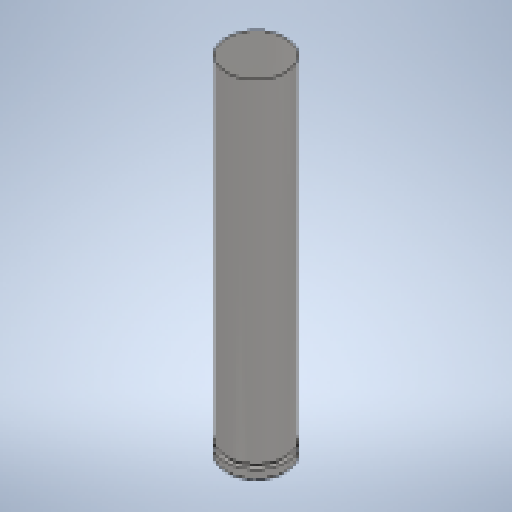
# Autodesk Inventor part: SHAFT
Saved by Autodesk Inventor 2023.2 (Build 272271000, 271)
## iProperties
Created: 2024-01-31
Part Number: SHAFT
Material: Stainless Steel
Document SubType Name: Modeling
Designer: Nathan Cai
Density: 8 g/cm^3
Appearance: Semi-Polished
Author: Nathan Cai
Autodesk Inventor part; units mm, degrees
ref_plane "YZ Plane" through (0, 0, 0) normal (1, 0, 0) x (0, 1, 0)
ref_plane "XZ Plane" through (0, 0, 0) normal (0, 1, 0) x (-1, 0, 0)
ref_plane "XY Plane" through (0, 0, 0) normal (0, 0, 1) x (1, 0, 0)
sketch "Sketch1" plane through (0, 0, 0) normal (0, 0, 1) x (1, 0, 0)
  line L0 (0, 0) -> (1.5, 0)
  line L1 (1.5, 0) -> (1.5, 18)
  line L2 (1.5, 18) -> (0, 18)
  line L3 (0, 18) -> (0, 0)
  line L4 (1.5, 0.5) -> (1.4, 0.5)
  line L5 (1.4, 0.5) -> (1.4, 1)
  line L6 (1.4, 1) -> (1.5, 1)
  line L7 (1.5, 1) -> (1.5, 0.5)
  point P0 (1.5, 1)
  dimension "d0" = 1.5
  dimension "d1" = 18
  dimension "d2" = 0.1
  dimension "d3" = 0.5
  dimension "d4" = 0.5
  constraints: 16 end point, 4 parallel, 2 horizontal, 2 perpendicular, 1 point on line
  measures "d0" distance of L2.end L1.end
  measures "d1" distance of L1.end L0.end
  measures "d2" distance of L5.end L6.end
  measures "d3" distance of L4.end L5.end
  measures "d4" distance between parallel lines of L0 L4
revolve "Revolution1" add sketch "Sketch1" angle 360 about axis through (0, 18, 0) along (0, -1, 0) contours L3 L2 L1 L6 L5 L4 L0
chamfer "Chamfer1" distance 0.1 angle 45 1 edges at (-1.5, 0, 0)
body "Solid1"
